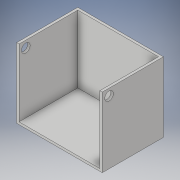
# Autodesk Inventor part: Collector V2
Saved by Autodesk Inventor 2019 (Build 230136000, 136)
## iProperties
Created: 2019-01-31
Part Number: Collector V2
Material: Generic
Document SubType Name: Modeling
Designer: Ashley
Density: 1 g/cm^3
Appearance: Default
Author: Ashley
Autodesk Inventor part; units mm, degrees
ref_plane "YZ Plane" through (0, 0, 0) normal (1, 0, 0) x (0, 1, 0)
ref_plane "XZ Plane" through (0, 0, 0) normal (0, 1, 0) x (-1, 0, 0)
ref_plane "XY Plane" through (0, 0, 0) normal (0, 0, 1) x (1, 0, 0)
sketch "Sketch1" plane through (0, 0, 0) normal (0, 1, 0) x (-1, 0, 0)
  line L0 (-70, -50) -> (70, -50)
  line L1 (70, -50) -> (70, 50)
  line L2 (70, 50) -> (-70, 50)
  line L3 (-70, 50) -> (-70, -50)
  line L4 (-70, -50) -> (70, 50) construction
  line L5 (70, -50) -> (-70, 50) construction
  point P0 (0, 0)
  dimension "d0" = 100
  dimension "d1" = 140
  constraints: 12 end point, 2 midpoint, 2 parallel, 1 horizontal, 1 perpendicular
  measures "d0" distance of L0.end L1.end
  measures "d1" distance of L0.start L0.end
extrude "Base Extrusion" add sketch "Sketch1" along normal blind 4
sketch "Sketch2" plane through (0, 4, 0) normal (0, 1, 0) x (1, 0, 0)
  line L0 (70, 50) -> (-70, 50) construction
  line L1 (-70, 50) -> (-70, -50) construction
  line L2 (-70, -50) -> (70, -50) construction
  line L3 (70, -50) -> (70, 50) construction
  line L4 (-70, 50) -> (70, 50)
  line L5 (70, 50) -> (70, 46)
  line L6 (70, 46) -> (-70, 46)
  line L7 (-70, 46) -> (-70, 50)
  line L8 (70, -50) -> (66, -50)
  line L9 (66, -50) -> (66, 50)
  line L10 (66, 50) -> (70, 50)
  line L11 (70, 50) -> (70, -50)
  line L12 (-70, 50) -> (-66, 50)
  line L13 (-66, 50) -> (-66, -50)
  line L14 (-66, -50) -> (-70, -50)
  line L15 (-70, -50) -> (-70, 50)
  point P0 (0, 0)
  dimension "d4" = 4
  dimension "d5" = 4
  dimension "d6" = 4
  constraints: 24 end point, 9 collinear, 6 parallel, 3 horizontal, 3 perpendicular
  measures "d4" distance between parallel lines of L0 L6
  measures "d5" distance between parallel lines of L1 L13
  measures "d6" distance between parallel lines of L3 L9
extrude "Height Extrusion" add sketch "Sketch2" along normal blind 110.075
sketch "Sketch3" plane through (70, 0, 50) normal (1, 0, 0) x (0, 0, -1)
  line L0 (0, 0) -> (0, 114.075) construction
  circle A0 centre (11.075, 103) radius 7.075
  point P0 (50, 0)
  dimension "d9" = 14.15
  dimension "d10" = 103
  dimension "d11" = 11.075
  constraints: 1 centre point
  measures "d9" diameter of A0
  measures "d10" vertical distance of point (50, 0) A0.centre
  measures "d11" distance from line of L0 A0.centre
extrude "Bearing Holes Cut" cut sketch "Sketch3" against normal up to surface (140 mm away)
equation "\"d0\" = BaseL"
equation "\"d1\" = BaseW"
equation "\"d2\" = uw"
equation "\"d4\" = uw"
equation "\"d5\" = uw"
equation "\"d6\" = uw"
equation "\"d7\" = Height"
equation "\"d9\" = BearingD"
equation "\"d10\" = AxelH + uw"
equation "\"d11\" = 0.5 * BearingD + uw"
equation "\"d12\" = Height"
equation "\"BallD\" = 76.2"
equation "\"BaseW\" = 140"
equation "\"BaseL\" = 100"
equation "\"AxelH\" = 99"
equation "\"Height\" = 0.5 * BearingD + AxelH + uw"
equation "\"BearingD\" = 14.15"
equation "\"uw\" = 4"
equation "\"ScrewD\" = 4.15"
equation "\"DistBtwnScrewandWall\" = 4"
equation "\"DistBtwnScrewHoles\" = 8"
body "Solid1"
